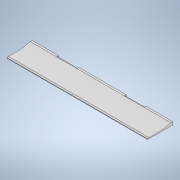
# Autodesk Inventor part: Pen Holder ReDes
Saved by Autodesk Inventor 2020.2 (Build 242310000, 310)
## iProperties
Created: 2020-05-07
Part Number: Pen Holder ReDes
Material: Generic
Document SubType Name: Modeling
Designer: Amaan Khalid
Density: 1 g/cm^3
Appearance: Default
Author: Amaan Khalid
Autodesk Inventor part; units mm, degrees
ref_plane "YZ Plane" through (0, 0, 0) normal (1, 0, 0) x (0, 1, 0)
ref_plane "XZ Plane" through (0, 0, 0) normal (0, 1, 0) x (-1, 0, 0)
ref_plane "XY Plane" through (0, 0, 0) normal (0, 0, 1) x (1, 0, 0)
sketch "Sketch1" plane through (0, 0, 0) normal (1, 0, 0) x (0, 1, 0)
  arc A0 (6.7804, 47.2423) -> (8.8296, 19.3623) centre (78.9029, 38.5279) ccw
  line L0 (5.5196, 48.6647) -> (5.1035, 48.6647)
  line L1 (5.1035, 48.6647) -> (5.1035, 16.8223)
  line L2 (5.1035, 16.8223) -> (8.8296, 16.8223)
  line L3 (8.8296, 16.8223) -> (8.8296, 19.3623)
  arc A1 (6.7804, 47.2423) -> (5.5196, 48.6647) centre (5.5196, 47.3947) ccw
  point P0 (0, 0)
  point P1 (6.9666, 48.6647)
  dimension "d0" = 1.27
  dimension "d1" = 2.54
  constraints: 8 end point, 5 point on circle, 2 centre point, 2 horizontal, 2 perpendicular, 2 tangent, 1 point on line
  measures "d0" radius of A1
  measures "d1" distance of L2.end L3.end
extrude "Extrusion1" add sketch "Sketch1" along normal blind 177.8
sketch "Sketch2" plane through (0, 8.8296, 19.3623) normal (0, 1, 0) x (1, 0, 0)
  line L0 (0, 0) -> (177.8, 0) projected
  line L1 (144.0688, 2.54) -> (144.0688, 0)
  line L2 (144.0688, 0) -> (118.6688, 0)
  line L3 (118.6688, 0) -> (118.6688, 2.54)
  line L4 (144.0688, 2.54) -> (118.6688, 2.54)
  line L5 (0, 2.54) -> (0, 0) projected
  line L6 (0, 1.27) -> (33.7312, 1.27)
  line L7 (0, 2.54) -> (177.8, 2.54) projected
  line L8 (33.7312, 2.54) -> (33.7312, 0)
  line L9 (33.7312, 0) -> (59.1312, 0)
  line L10 (59.1312, 0) -> (59.1312, 2.54)
  line L11 (59.1312, 2.54) -> (33.7312, 2.54)
  line L12 (177.8, 2.54) -> (177.8, 0) projected
  point P0 (0, 19.3623)
  dimension "d6" = 25.4
  dimension "d9" = 33.7312
  dimension "d10" = 25.4
  dimension "d11" = 2.54
  constraints: 18 end point, 5 point on line, 4 perpendicular, 1 horizontal, 1 midpoint
  measures "d6" distance of L1.end L2.end
  measures "d9" distance of L6.start L6.end
  measures "d10" distance of L8.end L9.end
  measures "d11" distance of L2.end L3.end
extrude "Extrusion2" cut sketch "Sketch2" against normal up to surface (1.863 mm away) contours L8 L7 L10 L0 | L3 L4 L1 L0
body "Solid1"
